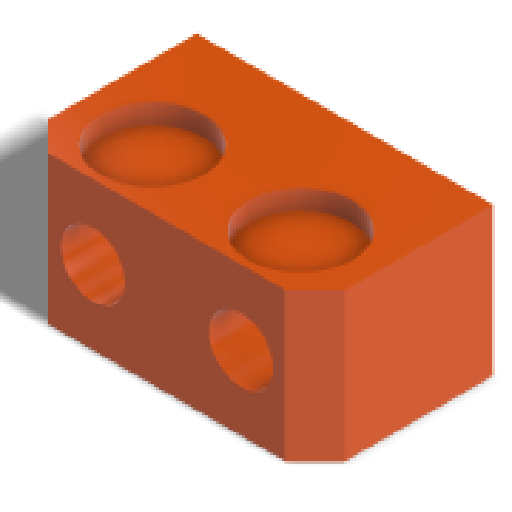
# Autodesk Inventor part: Door Base Magnet
Saved by Autodesk Inventor 2023.2 (Build 272271000, 271)
## iProperties
Created: 2023-03-04
Part Number: Door Base Magnet
Material: ABS Plastic
Document SubType Name: Modeling
Designer: remop
Density: 1.06 g/cm^3
Appearance: Smooth - Light Orange
Author: remop
Autodesk Inventor part; units mm, degrees
ref_plane "YZ Plane" through (0, 0, 0) normal (1, 0, 0) x (0, 1, 0)
ref_plane "XZ Plane" through (0, 0, 0) normal (0, 1, 0) x (-1, 0, 0)
ref_plane "XY Plane" through (0, 0, 0) normal (0, 0, 1) x (1, 0, 0)
sketch "Sketch1" plane through (0, 0, 0) normal (0, 0, 1) x (1, 0, 0)
  line L0 (15, -7.5) -> (-15, -7.5)
  line L1 (-15, -7.5) -> (-15, 7.5)
  line L2 (-15, 7.5) -> (15, 7.5)
  line L3 (15, 7.5) -> (15, -7.5)
  line L4 (15, -7.5) -> (-15, 7.5) construction
  line L5 (-15, -7.5) -> (15, 7.5) construction
  point P0 (0, 0)
  dimension "d0" = 15
  dimension "d1" = 30
  constraints: 12 end point, 2 midpoint, 2 parallel, 1 horizontal, 1 perpendicular
  measures "d0" distance of L0.end L1.end
  measures "d1" distance of L1.end L2.end
extrude "Extrusion1" add sketch "Sketch1" along normal blind 18
sketch "Sketch2" plane through (-15, 7.5, 0) normal (0, 1, 0) x (1, 0, 0)
  line L0 (30, 0) -> (0, 0) projected
  line L1 (0, 0) -> (0, -18) projected
  line L2 (30, -18) -> (0, -18) projected
  line L3 (30, 0) -> (30, -18) projected
  circle A0 centre (7.5, -12) radius 5.25
  circle A1 centre (22.5, -12) radius 5.25
  line L4 (30, 0) -> (0, 0) projected
  point P0 (15, 0)
  point P1 (15, 0)
  point P2 (15, 0)
  dimension "d4" = 10.5
  dimension "d5" = 6
  dimension "d6" = 7.5
  dimension "d7" = 7.5
  constraints: 2 centre point, 2 midpoint, 1 equal radius, 1 horizontal alignment
  measures "d4" diameter of A0
  measures "d5" distance from line of L2 A0.centre
  measures "d6" horizontal distance of point (15, 0) A0.centre
  measures "d7" horizontal distance of point (15, 0) A1.centre
extrude "Extrusion2" cut sketch "Sketch2" against normal blind 2 contours A0 | A1
chamfer "Chamfer1" distance 3 angle 45 2 edges at (15, 0, 18) (-15, 0, 18)
sketch "Sketch3" plane through (0, 0, 18) normal (0, 0, 1) x (1, 0, 0)
  line L0 (-12, -7.5) -> (-12, 7.5) projected
  line L1 (-12, -7.5) -> (12, -7.5) projected
  line L2 (12, 7.5) -> (12, -7.5) projected
  line L3 (12, 7.5) -> (-12, 7.5) projected
  point P0 (0, 0)
  point P1 (-7.5, 0)
  point P2 (7.5, 0)
  dimension "d13" = 7.5
  dimension "d14" = 7.5
  constraints: 2 horizontal alignment
  measures "d13" distance of point (-7.5, 0) point (0, 0)
  measures "d14" distance of point (7.5, 0) point (0, 0)
hole "Hole1" at (-7.5, 0, 18) at (7.5, 0, 18) direction (0, 0, -1) diameter 3.6 end through all counterbore diameter 6.5 counterbore depth 9 clearance for "Socket Head Cap Screw ISO 4762" size "M3" standard "ISO"
equation "\"d7\" = d6"
equation "\"d14\" = d13"
body "Solid1"
